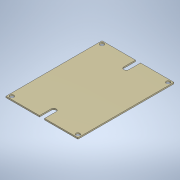
# Autodesk Inventor part: etl standard baseplate with cutouts
Saved by Autodesk Inventor 2022 (Build 260153000, 153)
## iProperties
Created: 2021-07-27
Part Number: etl standard baseplate with cutouts
Material: Generic
Document SubType Name: Modeling
Designer: Caleb
Density: 1 g/cm^3
Appearance: Default
Sending System: Autodesk Inventor 2022
Preprocessor: ST-DEVELOPER v18.1
Title: C:\Users\Caleb\Desktop\etl standard baseplate.stp
Author: Caleb
Autodesk Inventor part; units mm, degrees
ref_plane "YZ Plane" through (0, 0, 0) normal (1, 0, 0) x (0, 1, 0)
ref_plane "XZ Plane" through (0, 0, 0) normal (0, 1, 0) x (-1, 0, 0)
ref_plane "XY Plane" through (0, 0, 0) normal (0, 0, 1) x (1, 0, 0)
sketch "Sketch2" plane through (0, 0, 0) normal (0, 1, 0) x (-1, 0, 0)
  line L0 (-21.55, -28.75) -> (21.55, -28.75)
  line L1 (21.55, -28.75) -> (21.55, 28.75)
  line L2 (21.55, 28.75) -> (-21.55, 28.75)
  line L3 (-21.55, 28.75) -> (-21.55, -28.75)
  line L4 (-21.55, -28.75) -> (21.55, 28.75) construction
  line L5 (21.55, -28.75) -> (-21.55, 28.75) construction
  point P0 (0, 0)
  dimension "d28" = 43.1
  dimension "d29" = 57.5
  constraints: 12 end point, 2 midpoint, 2 parallel, 1 horizontal, 1 perpendicular
  measures "d28" distance of L1.end L2.end
  measures "d29" distance of L0.end L1.end
extrude "Extrusion2" add sketch "Sketch2" along normal blind 0.787
sketch "Sketch3" plane through (0, 0.787, 0) normal (0, 1, 0) x (1, 0, 0)
  line L0 (21.55, 28.75) -> (-21.55, 28.75) projected
  line L1 (3.17, 0) -> (-3.4256, 0) construction
  line L2 (-1.5, -28.75) -> (-1.5, -21.75)
  line L3 (1.5, -21.75) -> (1.5, -28.75)
  arc A0 (1.5, -21.75) -> (-1.5, -21.75) centre (0, -21.75) ccw
  line L4 (-21.55, -28.75) -> (21.55, -28.75) projected
  line L5 (-1.5, 28.75) -> (-1.5, 21.75)
  line L6 (1.5, 21.75) -> (1.5, 28.75)
  arc A1 (-1.5, 21.75) -> (1.5, 21.75) centre (0, 21.75) ccw
  line L7 (-21.55, 28.75) -> (21.55, 28.75)
  point P0 (0, 0)
  point P1 (1.5, 28.75)
  point P2 (-1.5, 28.75)
  dimension "d32" = 3
  dimension "d33" = 7
  dimension "d34" = 1.5
  constraints: 12 end point, 5 symmetric about line, 4 point on circle, 4 point on line, 2 centre point, 2 parallel, 1 horizontal, 1 perpendicular, 1 vertical alignment, 1 other
  measures "d32" distance between parallel lines of L2 L3
  measures "d33" distance of L2.start L2.end
  measures "d34" radius of A0
extrude "Extrusion3" cut sketch "Sketch3" against normal through all
sketch "Sketch4" plane through (0, 0.787, 0) normal (0, 1, 0) x (1, 0, 0)
  line L0 (-21.55, 28.75) -> (-21.55, -28.75) projected
  line L1 (-21.55, -28.75) -> (-1.5, -28.75) projected
  line L2 (21.55, -28.75) -> (21.55, 28.75) projected
  line L3 (-1.5, 28.75) -> (-21.55, 28.75) projected
  point P0 (0, 0)
  point P1 (-19.8, -27)
  point P2 (-19.8, 27)
  point P3 (19.8, -27)
  point P4 (19.8, 27)
  dimension "d37" = 1.75
  dimension "d38" = 1.75
  dimension "d39" = 1.75
  dimension "d40" = 1.75
  constraints: 2 horizontal alignment, 2 vertical alignment
  measures "d37" distance from line of L0 point (-19.8, -27)
  measures "d38" distance from line of L1 point (-19.8, -27)
  measures "d39" distance from line of L2 point (19.8, -27)
  measures "d40" distance from line of L3 point (-19.8, 27)
hole "Hole1" at (-19.8, 0.787, 27) at (-19.8, 0.787, -27) at (19.8, 0.787, 27) at (19.8, 0.787, -27) direction (0, -1, 0) diameter 2.4 end through all clearance for "Flat Head Machine Screw" size "M2" standard "Ansi Metric M Profile"
equation "\"d39\" = d37"
equation "\"d40\" = d38"
body "Solid3"
